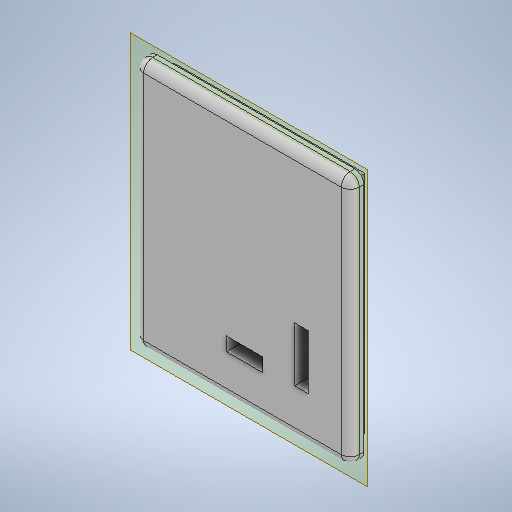
# Autodesk Inventor part: a4988_box_lid
Saved by Autodesk Inventor 2025 (Build 290162000, 162)
## iProperties
Created: 2025-03-03
Part Number: a4988_box_lid
Material: Všeobecné
Document SubType Name: Modeling
Designer: lukas
Density: 1 g/cm^3
Appearance: Výchozí
Author: lukas
## iProperties of the stored document a4988_box_lid_3D tisk.ipt
Created: 2025-03-03
Part Number: a4988_box_lid_3D tisk
Material: Všeobecné
Document SubType Name: Modeling
Designer: lukas
Density: 1 g/cm^3
Appearance: Výchozí
Author: lukas
Autodesk Inventor part; units mm, degrees
ref_plane "YZ Plane" through (0, 0, 0) normal (1, 0, 0) x (0, 1, 0)
ref_plane "XZ Plane" through (0, 0, 0) normal (0, 1, 0) x (-1, 0, 0)
sketch "Náčrt1" plane through (0, 0, 0) normal (0, 0, 1) x (1, 0, 0)
  line L0 (0, 35) -> (0, -35) projected
  line L1 (-29.75, 0) -> (29.75, 0) projected
  line L2 (21.25, -25) -> (-21.25, -25)
  line L3 (-21.25, -25) -> (-21.25, 25)
  line L4 (-21.25, 25) -> (21.25, 25)
  line L5 (21.25, 25) -> (21.25, -25)
  point P0 (0, 0)
  dimension "d0" = 42.5
  dimension "d1" = 50
  constraints: 8 end point, 2 parallel, 1 horizontal, 1 perpendicular, 2 other
  measures "d0" distance of L3.end L4.end
  measures "d1" distance of L4.end L2.start
extrude "Vysunutí1" add sketch "Náčrt1" along normal blind 3
sketch "Náčrt2" plane through (0, 0, 3) normal (0, 0, 1) x (1, 0, 0)
  line L0 (21.25, 25) -> (-21.25, 25) projected
  line L1 (-21.25, 25) -> (-21.25, -25) projected
  line L2 (-21.25, -25) -> (21.25, -25) projected
  line L3 (21.25, -25) -> (21.25, 25) projected
  line L4 (0, 35) -> (0, -35) projected
  line L5 (-29.75, 0) -> (29.75, 0) projected
  line L6 (4.5, -18.5) -> (-3.5, -18.5)
  line L7 (-3.5, -18.5) -> (-3.5, -15.5)
  line L8 (-3.5, -15.5) -> (4.5, -15.5)
  line L9 (4.5, -15.5) -> (4.5, -18.5)
  line L10 (14.5, -17.5) -> (11.5, -17.5)
  line L11 (11.5, -17.5) -> (11.5, -5.5)
  line L12 (11.5, -5.5) -> (14.5, -5.5)
  line L13 (14.5, -5.5) -> (14.5, -17.5)
  line L14 (-17.5, 21.5) -> (17.5, 21.5) construction
  line L15 (17.5, 21.5) -> (17.5, -21.5) construction
  line L16 (17.5, -21.5) -> (-17.5, -21.5) construction
  line L17 (-17.5, -21.5) -> (-17.5, 21.5) construction
  point P0 (0, 0)
  dimension "d4" = 12
  dimension "d5" = 3
  dimension "d6" = 8
  dimension "d7" = 3
  dimension "d9" = 35
  dimension "d10" = 43
  dimension "d11" = 3
  dimension "d13" = 3
  dimension "d29" = 16
  dimension "d30" = 21
  constraints: 24 end point, 6 parallel, 3 horizontal, 3 perpendicular, 2 other
  measures "d4" distance of L10.end L11.end
  measures "d5" distance of L11.end L12.end
  measures "d6" distance of L7.end L8.end
  measures "d7" distance of L8.end L6.start
  measures "d9" distance of L15.end L16.end
  measures "d10" distance between parallel lines of L16 L14
  measures "d11" distance between parallel lines of L6 L16
  measures "d13" distance between parallel lines of L15 L13
  measures "d29" distance between parallel lines of L16 L12
  measures "d30" distance between parallel lines of L15 L7
extrude "Vysunutí2" cut sketch "Náčrt2" against normal through all contours L8 L9 L6 L4 | L4 L6 L7 L8 | L10 L11 L12 L13
sketch "Náčrt3" plane through (0, 0, 3) normal (0, 0, 1) x (1, 0, 0)
  line L0 (-3.5, -18.5) -> (-3.5, -15.5) projected
  line L1 (-3.5, -15.5) -> (4.5, -15.5) projected
  line L2 (4.5, -15.5) -> (4.5, -18.5) projected
  line L3 (4.5, -18.5) -> (-3.5, -18.5) projected
  line L4 (11.5, -17.5) -> (11.5, -5.5) projected
  line L5 (11.5, -5.5) -> (14.5, -5.5) projected
  line L6 (14.5, -5.5) -> (14.5, -17.5) projected
  line L7 (14.5, -17.5) -> (11.5, -17.5) projected
  line L8 (21.25, 25) -> (-21.25, 25) projected
  line L9 (-21.25, 25) -> (-21.25, -25) projected
  line L10 (-21.25, -25) -> (21.25, -25) projected
  line L11 (21.25, -25) -> (21.25, 25) projected
  line L12 (0, 38.5) -> (0, -38.5) projected
  line L13 (-33.25, 0) -> (33.25, 0) projected
  line L14 (-19, 22.75) -> (19, 22.75)
  line L15 (19, 22.75) -> (19, -22.75)
  line L16 (19, -22.75) -> (-19, -22.75)
  line L17 (-19, -22.75) -> (-19, 22.75)
  line L18 (-21, 24.75) -> (21, 24.75)
  line L19 (21, 24.75) -> (21, -24.75)
  line L20 (21, -24.75) -> (-21, -24.75)
  line L21 (-21, -24.75) -> (-21, 24.75)
  point P0 (0, 0)
  dimension "d31" = 0.25
  dimension "d32" = 2
  constraints: 16 end point, 6 other
  measures "d31" distance between parallel lines of L8 L18
  measures "d32" distance between parallel lines of L18 L14
extrude "Vysunutí3" add sketch "Náčrt3" along normal blind 3 contours L16 L15 L13 L19 L20 L12 | L12 L20 L21 L13 L17 L16 | L14 L17 L13 L21 L18 L12 | L12 L18 L19 L13 L15 L14
sketch "Náčrt6" plane through (0, 0, 0) normal (0, 0, -1) x (-1, 0, 0)
  line L0 (3.5, -15.5) -> (3.5, -18.5) projected
  line L1 (3.5, -18.5) -> (-4.5, -18.5) projected
  line L2 (-4.5, -18.5) -> (-4.5, -15.5) projected
  line L3 (-4.5, -15.5) -> (3.5, -15.5) projected
  line L4 (-11.5, -5.5) -> (-11.5, -17.5) projected
  line L5 (-11.5, -17.5) -> (-14.5, -17.5) projected
  line L6 (-14.5, -17.5) -> (-14.5, -5.5) projected
  line L7 (-14.5, -5.5) -> (-11.5, -5.5) projected
  line L8 (-21.25, 25) -> (21.25, 25) projected
  line L9 (-21.25, -25) -> (-21.25, 25) projected
  line L10 (21.25, -25) -> (-21.25, -25) projected
  line L11 (21.25, 25) -> (21.25, -25) projected
  line L12 (0, -35) -> (0, 35) projected
  line L13 (-29.75, 0) -> (29.75, 0) projected
  line L14 (23.75, 27.5) -> (-23.75, 27.5)
  line L15 (-23.75, 27.5) -> (-23.75, -27.5)
  line L16 (-23.75, -27.5) -> (23.75, -27.5)
  line L17 (23.75, -27.5) -> (23.75, 27.5)
  point P0 (0, 0)
  dimension "d33" = 2.5
  constraints: 8 end point, 3 other
  measures "d33" distance between parallel lines of L8 L14
extrude "Vysunutí6" add sketch "Náčrt6" against normal up to surface (3 mm away) contours L12 L16 L15 L13 L9 L10 | L10 L11 L13 L17 L16 L12 | L12 L14 L17 L13 L11 L8 | L8 L9 L13 L15 L14 L12
ref_plane "Pracovní rovina1" through (0, 0, 1.5) normal (0, 0, -1) x (-1, 0, 0)
mirror "Zrcadlit1" about plane through (0, 0, 1.5) normal (0, 0, -1) of "Vysunutí3"
ref_plane "Pracovní rovina2" through (0, 0, 3) normal (0, 0, 1) x (1, 0, 0)
split "Rozdělit1" plane through (0, 0, 3) removes the side toward (0, 0, 1)
fillet "Zaoblení4" radius 2 8 edges at (23.75, 27.5, 1.5) (23.75, 0, 3) (0, 27.5, 3) (23.75, -27.5, 1.5) (0, -27.5, 3) (-23.75, 27.5, 1.5) (-23.75, 0, 3) (-23.75, -27.5, 1.5)
